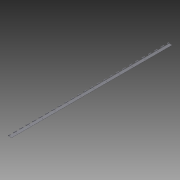
# Autodesk Inventor part: SIDE 1
Saved by Autodesk Inventor 2012 (Build 160160000, 160)
## iProperties
Created: 2015-09-17
Part Number: SIDE 1
Material: Steel, Mild
Document SubType Name: Modeling
Designer: testing
Density: 7.86 g/cm^3
Author: testing
Autodesk Inventor part; units mm, degrees
ref_plane "YZ Plane" through (0, 0, 0) normal (1, 0, 0) x (0, 1, 0)
ref_plane "XZ Plane" through (0, 0, 0) normal (0, 1, 0) x (-1, 0, 0)
ref_plane "XY Plane" through (0, 0, 0) normal (0, 0, 1) x (1, 0, 0)
sketch "Sketch2" plane through (0, 0, 0) normal (0, 1, 0) x (-1, 0, 0)
  arc A0 (0, -1.5) -> (-1.3365, -0.681) centre (0, 0) ccw
  arc A1 (0, -3) -> (-2.673, -1.362) centre (0, 0) ccw
  line L0 (0, -3) -> (-20, -3)
  line L1 (-20, -3) -> (-20, -1.5)
  line L2 (-20, -1.5) -> (0, -1.5)
  line L3 (-1.3365, -0.681) -> (-2.673, -1.362)
  dimension "d0" = 1.5
  dimension "d1" = 1.5
  dimension "d2" = 20
  dimension "d3" = 3
  dimension "d4" = 27
  constraints: 8 end point, 4 point on circle, 3 coincident, 2 centre point, 1 horizontal, 1 parallel, 1 perpendicular, 1 point on line, 1 tangent
  measures "d0" distance of L0.end L1.end
  measures "d1" radial gap between concentric circles of A1 A0
  measures "d2" distance from line of point (0, 0) L1
  measures "d3" diameter of A0
  measures "d4" angle of L2 L3
extrude "Extrusion1" add sketch "Sketch2" along normal blind 1000
sketch "Sketch3" plane through (20, 0, -3) normal (0, 0, -1) x (-1, 0, 0)
  line L0 (0, 0) -> (20, 0) projected
  line L1 (23, 30) -> (17, 30)
  line L2 (17, 30) -> (17, 10)
  line L3 (17, 10) -> (23, 10)
  line L4 (23, 10) -> (23, 30)
  line L5 (17, 0) -> (17, 1000) projected
  dimension "d7" = 10
  dimension "d8" = 20
  dimension "d9" = 6
  constraints: 8 end point, 2 parallel, 1 horizontal, 1 perpendicular, 1 point on line
  measures "d7" distance between parallel lines of L3 L0
  measures "d8" distance of L3.end L1.start
  measures "d9" distance of L2.end L3.end
extrude "Extrusion2" cut sketch "Sketch3" against normal through all
pattern_linear "Rectangular Pattern1" count 25 spacing 40 along (0, 1, 0) of "Extrusion2"
sketch "Sketch4" plane through (20, 0, -1.5) normal (0, 0, 1) x (1, 0, 0)
  line L0 (-20, 910) -> (-20, 930) projected
  line L1 (-20, 830) -> (-20, 850) projected
  line L2 (-20, 750) -> (-20, 770) projected
  line L3 (-20, 670) -> (-20, 690) projected
  line L4 (-20, 590) -> (-20, 610) projected
  line L5 (-20, 510) -> (-20, 530) projected
  line L6 (-20, 430) -> (-20, 450) projected
  line L7 (-20, 350) -> (-20, 370) projected
  line L8 (-20, 270) -> (-20, 290) projected
  line L9 (-20, 190) -> (-20, 210) projected
  line L10 (-20, 110) -> (-20, 130) projected
  line L11 (-20, 30) -> (-20, 50) projected
  line L12 (0, 0) -> (0, 1000) projected
  point P0 (-8, 40)
  point P1 (-8, 120)
  point P2 (-8, 200)
  point P3 (-8, 280)
  point P4 (-8, 360)
  point P5 (-8, 440)
  point P6 (-8, 520)
  point P7 (-8, 600)
  point P8 (-8, 680)
  point P9 (-8, 760)
  point P10 (-8, 840)
  point P11 (-8, 920)
  point P12 (-20, 40)
  point P13 (-20, 120)
  point P14 (-20, 200)
  point P15 (-20, 280)
  point P16 (-20, 360)
  point P17 (-20, 440)
  point P18 (-20, 520)
  point P19 (-20, 600)
  point P20 (-20, 680)
  point P21 (-20, 760)
  point P22 (-20, 840)
  point P23 (-20, 920)
  dimension "d15" = 8
  constraints: 12 horizontal alignment, 12 midpoint, 11 vertical alignment
  measures "d15" distance from line of L12 point (-8, 40)
hole "Hole1" at (12, 40, -1.5) at (12, 120, -1.5) at (12, 200, -1.5) at (12, 280, -1.5) at (12, 360, -1.5) at (12, 440, -1.5) at (12, 520, -1.5) at (12, 600, -1.5) at (12, 680, -1.5) at (12, 760, -1.5) at (12, 840, -1.5) at (12, 920, -1.5) direction (0, 0, -1) diameter 3 end through all countersink diameter 6 countersink angle 90
equation "\"d1\" = d0"
body "Solid1"
